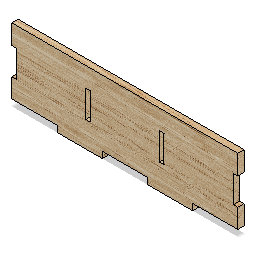
Assembly v13 (Autodesk Fusion 360 archive; units mm, degrees)
design "End"
Autodesk Fusion 360 part; units mm, degrees
sketch "Sketch1" plane through (0, 0, 0) normal (0, 0, 1) x (1, 0, 0)
  line L0 (0, 64) -> (200, 64)
  line L1 (200, 64) -> (200, 0)
  line L2 (200, 0) -> (0, 0)
  line L3 (0, 0) -> (0, 64)
  line L4 (0, 0) -> (40, 0)
  line L5 (40, 0) -> (40, 5.6)
  line L6 (40, 5.6) -> (0, 5.6)
  line L7 (0, 5.6) -> (0, 0)
  line L8 (80, 0) -> (120, 0)
  line L9 (120, 5.6) -> (80, 5.6)
  line L10 (120, 0) -> (120, 5.6)
  line L11 (80, 5.6) -> (80, 0)
  line L12 (160, 0) -> (200, 0)
  line L13 (200, 5.6) -> (160, 5.6)
  line L14 (200, 0) -> (200, 5.6)
  line L15 (160, 5.6) -> (160, 0)
  line L16 (0, 46.6) -> (3.95, 46.6)
  line L17 (3.95, 46.6) -> (3.95, 22.6)
  line L18 (3.95, 22.6) -> (0, 22.6)
  line L19 (0, 22.6) -> (0, 46.6)
  line L20 (69.3, 46.6) -> (69.3, 22.6)
  line L21 (65.35, 46.6) -> (69.3, 46.6)
  line L22 (65.35, 22.6) -> (65.35, 46.6)
  line L23 (69.3, 22.6) -> (65.35, 22.6)
  line L24 (134.65, 46.6) -> (134.65, 22.6)
  line L25 (130.7, 46.6) -> (134.65, 46.6)
  line L26 (130.7, 22.6) -> (130.7, 46.6)
  line L27 (134.65, 22.6) -> (130.7, 22.6)
  line L28 (200, 46.6) -> (200, 22.6)
  line L29 (196.05, 46.6) -> (200, 46.6)
  line L30 (196.05, 22.6) -> (196.05, 46.6)
  line L31 (200, 22.6) -> (196.05, 22.6)
  dimension "d84" = 64
  dimension "d85" = 200
  dimension "d93" = 40
  dimension "d94" = 5.6
  dimension "d97" = 160
  dimension "d98" = 0
  dimension "d105" = 3.95
  dimension "d106" = 24
  dimension "d108" = 17
  dimension "d123" = 196.05
  dimension "d124" = 0
  constraint horizontal L0
  constraint horizontal L2
  constraint horizontal L4
  constraint vertical L5
  constraint horizontal L6
  constraint vertical L7
  constraint coincident L2.end L3.start
  constraint horizontal L16
  constraint vertical L17
  constraint horizontal L18
  constraint vertical L19
  constraint coincident L3 L16.start
  constraint vertical L3
  measures "d84" distance of L0 L2
  measures "d85" distance of L1 L3
  measures "d93" distance of L2.end L4.end
  measures "d94" distance of L2.end L6.end
  measures "d105" distance of L17 L19
  measures "d106" distance of L16 L18
  measures "d108" distance of L6 L18
extrude "Extrude2" add sketch "Sketch1" along normal blind 5.6 contours L0 L1 L2 L3 L5 L6 L9 L10 L11 L13 L15 L16 L17 L18 L29 L30 L31
equation "kerf = 0.25 mm"
equation "d104 = 13.25 mm - kerf"

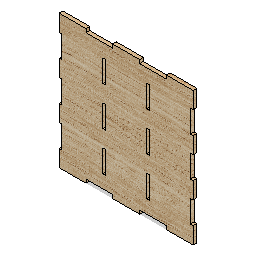
design "Bottom"
Autodesk Fusion 360 part; units mm, degrees
sketch "Sketch1" plane through (0, 0, 0) normal (0, 0, 1) x (1, 0, 0)
  line L0 (0, 0) -> (200, 0)
  line L1 (200, 0) -> (200, 200)
  line L2 (200, 200) -> (0, 200)
  line L3 (0, 200) -> (0, 0)
  line L4 (40.1, 0) -> (79.9, 0)
  line L5 (79.9, 0) -> (79.9, 5.3)
  line L6 (79.9, 5.3) -> (40.1, 5.3)
  line L7 (40.1, 5.3) -> (40.1, 0)
  line L8 (159.9, 0) -> (159.9, 5.3)
  line L9 (159.9, 5.3) -> (120.1, 5.3)
  line L10 (120.1, 5.3) -> (120.1, 0)
  line L11 (120.1, 0) -> (159.9, 0)
  line L12 (79.9, 194.7) -> (79.9, 200)
  line L13 (79.9, 200) -> (40.1, 200)
  line L14 (40.1, 200) -> (40.1, 194.7)
  line L15 (40.1, 194.7) -> (79.9, 194.7)
  line L16 (159.9, 194.7) -> (159.9, 200)
  line L17 (159.9, 200) -> (120.1, 200)
  line L18 (120.1, 200) -> (120.1, 194.7)
  line L19 (120.1, 194.7) -> (159.9, 194.7)
  line L20 (0, 175) -> (4.05, 175)
  line L21 (4.05, 175) -> (4.05, 141.67)
  line L22 (4.05, 141.67) -> (0, 141.67)
  line L23 (0, 141.67) -> (0, 175)
  line L24 (65.3167, 175) -> (69.3667, 175)
  line L25 (69.3667, 141.67) -> (65.3167, 141.67)
  line L26 (65.3167, 141.67) -> (65.3167, 175)
  line L27 (69.3667, 175) -> (69.3667, 141.67)
  line L28 (130.6333, 175) -> (134.6833, 175)
  line L29 (134.6833, 141.67) -> (130.6333, 141.67)
  line L30 (130.6333, 141.67) -> (130.6333, 175)
  line L31 (134.6833, 175) -> (134.6833, 141.67)
  line L32 (195.95, 175) -> (200, 175)
  line L33 (200, 141.67) -> (195.95, 141.67)
  line L34 (195.95, 141.67) -> (195.95, 175)
  line L35 (200, 175) -> (200, 141.67)
  line L36 (0, 116.665) -> (4.05, 116.665)
  line L37 (4.05, 83.335) -> (0, 83.335)
  line L38 (0, 83.335) -> (0, 116.665)
  line L39 (4.05, 116.665) -> (4.05, 83.335)
  line L40 (65.3167, 116.665) -> (69.3667, 116.665)
  line L41 (69.3667, 83.335) -> (65.3167, 83.335)
  line L42 (65.3167, 83.335) -> (65.3167, 116.665)
  line L43 (69.3667, 116.665) -> (69.3667, 83.335)
  line L44 (130.6333, 116.665) -> (134.6833, 116.665)
  line L45 (134.6833, 83.335) -> (130.6333, 83.335)
  line L46 (130.6333, 83.335) -> (130.6333, 116.665)
  line L47 (134.6833, 116.665) -> (134.6833, 83.335)
  line L48 (195.95, 116.665) -> (200, 116.665)
  line L49 (200, 83.335) -> (195.95, 83.335)
  line L50 (195.95, 83.335) -> (195.95, 116.665)
  line L51 (200, 116.665) -> (200, 83.335)
  line L52 (0, 58.33) -> (4.05, 58.33)
  line L53 (4.05, 25) -> (0, 25)
  line L54 (0, 25) -> (0, 58.33)
  line L55 (4.05, 58.33) -> (4.05, 25)
  line L56 (65.3167, 58.33) -> (69.3667, 58.33)
  line L57 (69.3667, 25) -> (65.3167, 25)
  line L58 (65.3167, 25) -> (65.3167, 58.33)
  line L59 (69.3667, 58.33) -> (69.3667, 25)
  line L60 (130.6333, 58.33) -> (134.6833, 58.33)
  line L61 (134.6833, 25) -> (130.6333, 25)
  line L62 (130.6333, 25) -> (130.6333, 58.33)
  line L63 (134.6833, 58.33) -> (134.6833, 25)
  line L64 (195.95, 58.33) -> (200, 58.33)
  line L65 (200, 25) -> (195.95, 25)
  line L66 (195.95, 25) -> (195.95, 58.33)
  line L67 (200, 58.33) -> (200, 25)
  dimension "d15" = 200
  dimension "d16" = 200
  dimension "d23" = 39.8
  dimension "d24" = 5.3
  dimension "d25" = 40.1
  dimension "d28" = 80
  dimension "d29" = 194.7
  dimension "d30" = 4.05
  dimension "d31" = 33.33
  dimension "d32" = 25
  dimension "d35" = 195.95
  dimension "d36" = -116.67
  constraint vertical L1
  constraint vertical L3
  constraint coincident L0.start L3.end
  constraint horizontal L4
  constraint vertical L5
  constraint horizontal L6
  constraint vertical L7
  constraint coincident L0 L4.start
  constraint horizontal L20
  constraint vertical L21
  constraint horizontal L22
  constraint vertical L23
  constraint coincident L3 L20.start
  measures "d15" distance of L0.start L0.end
  measures "d16" distance of L0.start L2.end
  measures "d23" distance of L4.start L4.end
  measures "d24" distance of L4.start L6.end
  measures "d25" distance of L3 L7
  measures "d30" distance of L20.start L20.end
  measures "d31" distance of L20.start L22.end
  measures "d32" distance of L2 L20
extrude "Extrude1" add sketch "Sketch1" along normal blind 5.6 contours L0 L1 L2 L3 L5 L6 L7 L8 L9 L10 L12 L14 L15 L16 L18 L19 L20 L21 L22 L32 L33 L34 L36 L37 L39 L48 L49 L50 L52 L53 L55 L64 L65 L66
equation "kerf = 0.25 mm"

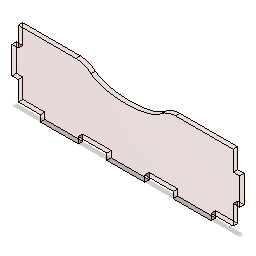
design "Side"
Autodesk Fusion 360 part; units mm, degrees
sketch "Sketch1" plane through (0, 0, 0) normal (0, 0, 1) x (1, 0, 0)
  line L0 (0, 64) -> (200, 64)
  line L1 (200, 0) -> (0, 0)
  line L2 (0, 0) -> (25, 0)
  line L3 (25, 0) -> (25, 5.6)
  line L4 (25, 5.6) -> (0, 5.6)
  line L5 (66.667, 69) -> (66.667, 59) construction
  line L6 (100, 73.2587) -> (100, 54.7413)
  ellipse E0 centre (100, 64) end of major axis (66.667, 64) minor radius 12.5
  line L7 (133.333, 64) -> (66.667, 64)
  line L8 (100, 76.5) -> (100, 51.5)
  line L9 (0, 64) -> (0, 0)
  line L10 (5.6, 64) -> (5.6, 5.6)
  line L11 (0, 46.6) -> (5.6, 46.6)
  line L12 (5.6, 46.6) -> (5.6, 22.6)
  line L13 (5.6, 22.6) -> (0, 22.6)
  line L14 (0, 22.6) -> (0, 46.6)
  line L15 (200, 64) -> (200, 0)
  line L16 (0, 5.6) -> (0, 0)
  line L17 (194.4, 64) -> (194.4, 5.6)
  line L18 (194.4, 46.6) -> (200, 46.6)
  line L19 (200, 46.6) -> (200, 22.6)
  line L20 (200, 22.6) -> (194.4, 22.6)
  line L21 (194.4, 22.6) -> (194.4, 46.6)
  line L22 (58.3333, 0) -> (83.3333, 0)
  line L23 (58.3333, 5.6) -> (58.3333, 0)
  line L24 (83.3333, 5.6) -> (58.3333, 5.6)
  line L25 (83.3333, 0) -> (83.3333, 5.6)
  line L26 (116.6667, 0) -> (141.6667, 0)
  line L27 (116.6667, 5.6) -> (116.6667, 0)
  line L28 (141.6667, 5.6) -> (116.6667, 5.6)
  line L29 (141.6667, 0) -> (141.6667, 5.6)
  line L30 (175, 0) -> (200, 0)
  line L31 (175, 5.6) -> (175, 0)
  line L32 (200, 5.6) -> (175, 5.6)
  line L33 (200, 0) -> (200, 5.6)
  point P0 (58.3333, 0)
  point P1 (58.3333, 0)
  point P2 (116.6667, 0)
  point P3 (116.6667, 0)
  point P4 (175, 0)
  point P5 (175, 0)
  dimension "d78" = 200
  dimension "d79" = 64
  dimension "d88" = 25
  dimension "d100" = 10
  dimension "d101" = 5
  dimension "d102" = 25
  dimension "d105" = 5.6
  dimension "d106" = 5.6
  dimension "d107" = 24
  dimension "d108" = 17
  dimension "d109" = 5.6
  dimension "d110" = 24
  dimension "d112" = 5.6
  dimension "d128" = 17
  dimension "d129" = 5.6
  dimension "d130" = 5.6
  dimension "d131" = 5.6
  constraint horizontal L0
  constraint horizontal L2
  constraint vertical L3
  constraint horizontal L4
  constraint coincident L1 L2.start
  constraint coincident L1.end L2.start
  constraint perpendicular L0 L6
  constraint midpoint L0 L6
  constraint midpoint L6 E0.centre
  constraint perpendicular L5 L7
  constraint coincident E0 L7.start
  constraint coincident E0 L7.end
  constraint coincident E0 L8.start
  constraint coincident E0 L8.end
  constraint perpendicular L1 L9
  constraint coincident L0 L10.start
  constraint coincident L4 L10.end
  constraint perpendicular L4 L10
  constraint horizontal L11
  constraint vertical L12
  constraint horizontal L13
  constraint vertical L14
  constraint coincident L9 L11.start
  constraint perpendicular L1 L16
  constraint coincident L0 L17.start
  constraint horizontal L18
  constraint vertical L19
  constraint horizontal L20
  constraint vertical L21
  constraint coincident L17 L18.start
  constraint vertical L15
  constraint coincident L17.end L32
  constraint perpendicular L17 L32
  constraint coincident L15 L18.end
  measures "d78" distance of L0.start L0.end
  measures "d79" distance of L0.start L1.end
  measures "d88" distance of L1.end L2.end
  measures "d100" distance of L5.start L5.end
  measures "d101" distance of L0 L5.start
  measures "d105" distance of L9 L10
  measures "d106" distance of L11.start L11.end
  measures "d107" distance of L11.start L13.end
  measures "d108" distance of L4 L13
  measures "d109" distance of L15 L17
  measures "d110" distance of L18.start L20.end
  measures "d112" distance of L1 L4
  measures "d128" distance of L20 L32
  measures "d129" distance of L1 L32
  measures "d130" distance of L22 L24
  measures "d131" distance of L26 L28
extrude "Extrude2" add sketch "Sketch1" along normal blind 3.9 contours L0 L1 L3 L4 E0 L10 L12 L17 L21 L23 L24 L25 L27 L28 L29 L31 L32 | L9 L10 L11 L12 L13 L14 | L15 L17 L18 L19 L20 L21
fillet "Fillet2" radius 20 2 edges at (66.667, 64, 1.95) (133.333, 64, 1.95)
